Autodesk Inventor part; units mm, degrees
note: some values were not read from the file. Chosen so that the rebuilt part matches the saved one: direction of "Hole2".
(part 2 of 20)
  ellipse E76 centre (-10075.27878, -10011.578305) end of major axis (-10075.513001, -10009.501471) minor radius 0.044517 (-10075.516592, -10009.569699) -> (-10075.486251, -10009.995005) ccw
  ellipse E77 centre (-10074.384652, -10011.477467) end of major axis (-10074.618874, -10009.400632) minor radius 0.044517 (-10074.622381, -10009.471498) -> (-10074.592437, -10009.890575) ccw
  ellipse E78 centre (-10060.476, -10009.908873) end of major axis (-10060.386346, -10010.703833) minor radius 0.01704 (-10060.484477, -10009.985098) -> (-10060.393632, -10010.678018) ccw
  line L94 (-10060.377876, -10010.91364) -> (-10060.484477, -10009.985098)
  ellipse E79 centre (-10059.482525, -10009.79683) end of major axis (-10059.426491, -10010.29368) minor radius 0.01065 (-10059.539194, -10009.3223) -> (-10059.42924, -10010.286086) ccw
  line L95 (-10062.350001, -10017.517567) -> (-10062.806719, -10017.467871)
  line L96 (-10060.454278, -10015.430074) -> (-10060.460552, -10016.580748)
  line L97 (-10059.880259, -10016.422198) -> (-10059.873105, -10015.110144)
  line L98 (-10059.873105, -10015.110144) -> (-10060.046355, -10015.004028)
  ellipse E80 centre (-10060.050028, -10015.677678) end of major axis (-10060.234317, -10014.96604) minor radius 0.371687 (-10060.442629, -10015.281983) -> (-10060.454278, -10015.430074) ccw
  ellipse E81 centre (-10060.050028, -10015.677678) end of major axis (-10060.234317, -10014.96604) minor radius 0.371687 (-10060.046355, -10015.004028) -> (-10060.05419, -10014.999356) ccw
  ellipse E82 centre (-10059.335003, -10016.824224) end of major axis (-10059.248465, -10016.028918) minor radius 0.273562 (-10059.101399, -10016.209395) -> (-10059.155812, -10016.093674) ccw
  line L99 (-10062.350001, -10020.512649) -> (-10062.806719, -10020.562345)
  ellipse E83 centre (-10060.025424, -10022.372531) end of major axis (-10059.932235, -10021.66476) minor radius 0.400382 (-10060.431835, -10022.539755) -> (-10059.992436, -10023.062247) ccw
  line L100 (-10060.063938, -10023.080853) -> (-10060.204432, -10023.096141)
  line L101 (-10060.476356, -10021.608916) -> (-10060.431835, -10022.539755)
  line L102 (-10059.992436, -10023.062247) -> (-10059.81826, -10022.990579)
  line L103 (-10059.81826, -10022.990579) -> (-10059.876504, -10021.77281)
  ellipse E84 centre (-10059.335003, -10021.369758) end of major axis (-10059.248465, -10022.165063) minor radius 0.273562 (-10059.155812, -10022.100307) -> (-10059.101399, -10021.984587) ccw
  ellipse E85 centre (-10061.469475, -10028.173067) end of major axis (-10061.55913, -10028.968027) minor radius 0.01704 (-10061.487267, -10028.178778) -> (-10061.56071, -10028.955341) ccw
  line L104 (-10061.487267, -10028.178778) -> (-10061.380198, -10027.227663)
  ellipse E86 centre (-10059.482525, -10028.397152) end of major axis (-10059.57218, -10029.192112) minor radius 0.01704 (-10059.407624, -10027.670855) -> (-10059.57111, -10029.119451) ccw
  line L105 (-10061.56497, -10026.585239) -> (-10062.078212, -10026.527356)
  ellipse E87 centre (-10075.27878, -10026.615677) end of major axis (-10075.513001, -10028.692511) minor radius 0.044517 (-10075.486251, -10028.198976) -> (-10075.513001, -10028.692511) ccw
  ellipse E88 centre (-10074.384652, -10026.716515) end of major axis (-10074.618874, -10028.793349) minor radius 0.044517 (-10074.592437, -10028.303407) -> (-10074.622381, -10028.722483) ccw
  line L106 (-10060.493792, -10028.290821) -> (-10060.380028, -10027.280229)
  ellipse E89 centre (-10060.476, -10028.285109) end of major axis (-10060.386346, -10027.490149) minor radius 0.01704 (-10060.393632, -10027.515964) -> (-10060.493792, -10028.290821) ccw
  ellipse E90 centre (-10059.482525, -10028.397152) end of major axis (-10059.538559, -10028.894002) minor radius 0.01065 (-10059.427694, -10027.953575) -> (-10059.528515, -10028.845931) ccw
  line L107 (-10061.48836, -10025.278009) -> (-10061.55116, -10026.262694)
  ellipse E91 centre (-10061.350908, -10025.73615) end of major axis (-10061.516786, -10026.518764) minor radius 0.120739 (-10061.55116, -10026.262694) -> (-10061.250304, -10025.840771) ccw
  line L108 (-10061.250304, -10025.840771) -> (-10060.901774, -10024.313165)
  line L109 (-10060.901774, -10024.313165) -> (-10059.934712, -10024.518137)
  ellipse E92 centre (-10059.416785, -10026.146094) end of major axis (-10059.582663, -10026.928708) minor radius 0.120739 (-10059.515377, -10026.862757) -> (-10059.215803, -10025.454922) ccw
  line L110 (-10061.508918, -10026.520431) -> (-10061.516786, -10026.518764)
  line L111 (-10060.925141, -10024.345935) -> (-10060.901774, -10024.313165)
  line L112 (-10060.901774, -10024.313165) -> (-10064.091636, -10023.637063)
  ellipse E93 centre (-10060.325762, -10024.379903) end of major axis (-10060.884685, -10023.567598) minor radius 0.235923 (-10060.180568, -10024.176282) -> (-10060.792125, -10023.567877) ccw
  line L113 (-10061.100929, -10023.500053) -> (-10067.010154, -10022.247573)
  line L114 (-10060.180568, -10024.176282) -> (-10059.934712, -10024.518137)
  line L115 (-10060.283242, -10026.045743) -> (-10059.934712, -10024.518137)
  line L116 (-10061.422518, -10013.14956) -> (-10061.856897, -10013.172389)
  line L117 (-10061.836081, -10012.326253) -> (-10061.553929, -10012.311424)
  line L118 (-10061.409576, -10013.39483) -> (-10061.492385, -10011.825491)
  ellipse E94 centre (-10061.492555, -10011.773328) end of major axis (-10061.534542, -10010.97443) minor radius 0.002573 (-10061.534542, -10010.97443) -> (-10061.492385, -10011.825491) ccw
  line L119 (-10061.36027, -10013.392238) -> (-10061.409576, -10013.39483)
  ellipse E95 centre (-10059.495322, -10011.66836) end of major axis (-10059.537309, -10010.869463) minor radius 0.002573 (-10059.510196, -10011.340621) -> (-10059.515377, -10011.331224) ccw
  line L120 (-10059.537309, -10010.869463) -> (-10061.534542, -10010.97443)
  line L121 (-10061.557698, -10012.065672) -> (-10061.853507, -10012.081219)
  line L122 (-10061.409576, -10013.39483) -> (-10063.048629, -10013.480972)
  ellipse E96 centre (-10059.495322, -10011.66836) end of major axis (-10059.521564, -10011.169049) minor radius 0.001608 (-10059.511461, -10011.338287) -> (-10059.514117, -10011.333468) ccw
  line L123 (-10061.607405, -10010.674865) -> (-10061.68528, -10010.670928)
  line L124 (-10061.783035, -10009.753857) -> (-10061.579243, -10009.76416)
  line L125 (-10061.615601, -10010.939927) -> (-10061.567206, -10009.374897)
  ellipse E97 centre (-10061.420853, -10009.294962) end of major axis (-10061.380459, -10008.495982) minor radius 0.142983 (-10061.380459, -10008.495982) -> (-10061.54092, -10009.012282) ccw
  line L126 (-10061.570957, -10010.942184) -> (-10061.615601, -10010.939927)
  ellipse E98 centre (-10059.455566, -10009.394321) end of major axis (-10059.415172, -10008.595341) minor radius 0.142983 (-10059.342552, -10008.734438) -> (-10059.57111, -10009.07453) ccw
  line L127 (-10059.415172, -10008.595341) -> (-10061.380459, -10008.495982)
  line L128 (-10061.571047, -10009.499098) -> (-10061.816602, -10009.486684)
  line L129 (-10061.615601, -10010.939927) -> (-10061.811814, -10010.930007)
  line L130 (-10063.391932, -10010.850121) -> (-10063.642743, -10010.837441)
  ellipse E99 centre (-10075.079596, -10008.604419) end of major axis (-10074.974067, -10006.517085) minor radius 0.373543 (-10074.974067, -10006.517085) -> (-10075.402988, -10007.952487) ccw
  ellipse E100 centre (-10074.195217, -10008.64913) end of major axis (-10074.089688, -10006.561796) minor radius 0.373543 (-10073.894561, -10006.951244) -> (-10074.51733, -10007.985402) ccw
  line L131 (-10074.974067, -10006.517085) -> (-10074.089688, -10006.561796)
  ellipse E101 centre (-10074.195217, -10008.64913) end of major axis (-10074.119478, -10007.151044) minor radius 0.268093 (-10074.014581, -10007.29359) -> (-10074.41067, -10009.869338) ccw
  ellipse E102 centre (-10059.455566, -10009.394321) end of major axis (-10059.43032, -10008.894959) minor radius 0.089364 (-10059.363417, -10009.208737) -> (-10059.544237, -10009.378772) ccw
  line L132 (-10059.898881, -10015.094356) -> (-10059.801569, -10014.609349)
  line L133 (-10059.801569, -10014.609349) -> (-10059.814039, -10014.600069)
  ellipse E103 centre (-10059.377353, -10016.449287) end of major axis (-10059.172257, -10015.676024) minor radius 0.142054 (-10059.155812, -10016.093674) -> (-10059.172257, -10015.676024) ccw
  line L134 (-10059.172257, -10015.676024) -> (-10059.875174, -10015.489586)
  line L135 (-10062.350001, -10019.545608) -> (-10062.806719, -10019.51725)
  line L136 (-10060.391402, -10027.491423) -> (-10060.332323, -10027.282736)
  ellipse E104 centre (-10060.305787, -10027.725657) end of major axis (-10060.527432, -10028.49434) minor radius 0.14613 (-10060.307433, -10027.284044) -> (-10060.393632, -10027.515964) ccw
  ellipse E105 centre (-10059.361099, -10027.998052) end of major axis (-10059.222572, -10027.517625) minor radius 0.091331 (-10059.227286, -10027.838895) -> (-10059.44944, -10027.974778) ccw
  ellipse E106 centre (-10059.361099, -10027.998052) end of major axis (-10059.139455, -10027.229369) minor radius 0.14613 (-10059.144207, -10027.729902) -> (-10059.407624, -10027.670855) ccw
  line L137 (-10059.139455, -10027.229369) -> (-10059.524741, -10027.118274)
  ellipse E107 centre (-10061.194651, -10025.032179) end of major axis (-10061.48409, -10025.777984) minor radius 0.002457 (-10061.46407, -10025.723867) -> (-10061.48409, -10025.777984) ccw
  ellipse E108 centre (-10061.194651, -10025.032179) end of major axis (-10060.905212, -10024.286374) minor radius 0.002457 (-10061.457945, -10025.707747) -> (-10061.458801, -10025.709998) ccw
  line L138 (-10060.660115, -10023.646866) -> (-10060.655933, -10023.636082)
  line L139 (-10060.655933, -10023.636082) -> (-10059.723681, -10023.997878)
  ellipse E109 centre (-10059.330147, -10025.755773) end of major axis (-10059.040708, -10025.009968) minor radius 0.002457 (-10059.21498, -10025.465271) -> (-10059.215803, -10025.454922) ccw
  line L140 (-10061.474672, -10025.781639) -> (-10061.48409, -10025.777984)
  line L141 (-10059.040708, -10025.009968) -> (-10059.965078, -10024.65123)
  line L142 (-10060.655933, -10023.636082) -> (-10060.696511, -10023.620334)
  line L143 (-10060.883309, -10023.547839) -> (-10065.815027, -10021.633895)
  ellipse E110 centre (-10059.984852, -10023.848112) end of major axis (-10060.377627, -10022.955787) minor radius 0.168714 (-10059.900944, -10023.626312) -> (-10060.345585, -10022.957249) ccw
  line L144 (-10060.345585, -10022.957249) -> (-10064.606408, -10021.303671)
  line L145 (-10059.900944, -10023.626312) -> (-10059.723681, -10023.997878)
  line L146 (-10059.723681, -10023.997878) -> (-10059.956311, -10024.612802)
  line L147 (-10059.947993, -10024.576347) -> (-10059.723681, -10023.997878)
  ellipse E111 centre (-10059.330147, -10025.755773) end of major axis (-10059.149248, -10025.289644) minor radius 0.001536 (-10059.215161, -10025.462782) -> (-10059.215594, -10025.457336) ccw
  line L148 (-10061.167264, -10013.708989) -> (-10061.411584, -10012.430812)
  ellipse E112 centre (-10061.419075, -10012.379718) end of major axis (-10061.569131, -10011.593917) minor radius 0.002231 (-10061.449697, -10012.231033) -> (-10061.411584, -10012.430812) ccw
  ellipse E113 centre (-10061.419075, -10012.379718) end of major axis (-10061.569131, -10011.593917) minor radius 0.002231 (-10061.569131, -10011.593917) -> (-10061.479166, -10012.076002) ccw
  line L149 (-10061.562628, -10011.592675) -> (-10061.569131, -10011.593917)
  line L150 (-10061.435333, -10010.969216) -> (-10061.540297, -10010.029174)
  ellipse E114 centre (-10074.188288, -10011.200402) end of major axis (-10074.334497, -10009.707545) minor radius 0.24157 (-10074.395592, -10009.772988) -> (-10074.425568, -10009.871079) ccw
  ellipse E115 centre (-10074.188288, -10011.200402) end of major axis (-10074.392006, -10009.120355) minor radius 0.336587 (-10074.468892, -10009.193821) -> (-10074.4718, -10009.199795) ccw
  ellipse E116 centre (-10059.45458, -10009.7574) end of major axis (-10059.405844, -10010.255019) minor radius 0.080523 (-10059.453007, -10010.190813) -> (-10059.427468, -10010.241126) ccw
  ellipse E117 centre (-10059.45458, -10009.7574) end of major axis (-10059.503316, -10009.259781) minor radius 0.080523 (-10059.517481, -10009.270082) -> (-10059.543695, -10009.384211) ccw
  ellipse E118 centre (-10061.390902, -10025.808057) end of major axis (-10061.238841, -10025.022641) minor radius 0.086818 (-10061.489391, -10025.861843) -> (-10061.564797, -10026.455678) ccw
  line L151 (-10061.489391, -10025.861843) -> (-10061.456687, -10025.683636)
  line L152 (-10061.230363, -10013.101701) -> (-10061.302045, -10012.860155)
  ellipse E119 centre (-10061.313455, -10012.81413) end of major axis (-10061.540932, -10012.047152) minor radius 0.002152 (-10061.359155, -10012.66747) -> (-10061.302045, -10012.860155) ccw
  ellipse E120 centre (-10061.313455, -10012.81413) end of major axis (-10061.540932, -10012.047152) minor radius 0.002152 (-10061.380234, -10012.596226) -> (-10061.379475, -10012.598795) ccw
  ellipse E121 centre (-10061.313455, -10012.81413) end of major axis (-10061.540932, -10012.047152) minor radius 0.002152 (-10061.540854, -10012.047696) -> (-10061.46729, -10012.301069) ccw
  line L153 (-10059.896065, -10014.082947) -> (-10060.229072, -10014.181713)
  line L154 (-10067.429747, -10016.109617) -> (-10067.426808, -10016.11971)
  line L155 (-10064.222927, -10015.366245) -> (-10067.081482, -10016.214061)
  line L156 (-10059.899344, -10014.071686) -> (-10059.896065, -10014.082947)
  line L157 (-10059.896065, -10014.082947) -> (-10059.936009, -10014.146629)
  line L158 (-10059.896065, -10014.082947) -> (-10059.964617, -10013.851948)
  line L159 (-10061.459654, -10010.510742) -> (-10061.463483, -10010.493181)
  ellipse E122 centre (-10061.347946, -10010.418573) end of major axis (-10061.510562, -10009.635275) minor radius 0.128538 (-10061.5089, -10010.257445) -> (-10061.463483, -10010.493181) ccw
  line L160 (-10060.361849, -10010.912798) -> (-10060.37563, -10010.849592)
  ellipse E123 centre (-10059.415142, -10010.017314) end of major axis (-10059.313507, -10010.506876) minor radius 0.080336 (-10059.449748, -10010.21676) -> (-10059.286923, -10010.372283) ccw
  ellipse E124 centre (-10061.442823, -10028.705225) end of major axis (-10061.437551, -10029.505207) minor radius 0.125799 (-10061.568714, -10028.685033) -> (-10061.437551, -10029.505207) ccw
  line L161 (-10061.568714, -10028.685033) -> (-10061.570469, -10027.970396)
  line L162 (-10061.572527, -10027.132339) -> (-10061.572581, -10027.110703)
  line L163 (-10061.572581, -10027.110703) -> (-10061.543326, -10027.110511)
  ellipse E125 centre (-10059.467748, -10028.69221) end of major axis (-10059.462476, -10029.492193) minor radius 0.125799 (-10059.587131, -10028.407305) -> (-10059.593638, -10028.672019) ccw
  line L164 (-10061.572581, -10027.110703) -> (-10062.110288, -10027.114246)
  line L165 (-10063.114705, -10027.120865) -> (-10063.630156, -10027.124262)
  ellipse E126 centre (-10075.169596, -10028.795676) end of major axis (-10075.155825, -10030.885631) minor radius 0.328649 (-10075.496217, -10028.957967) -> (-10075.432006, -10029.986721) ccw
  ellipse E127 centre (-10074.280812, -10028.789819) end of major axis (-10074.267041, -10030.879774) minor radius 0.328649 (-10074.605637, -10029.03444) -> (-10074.544121, -10029.973038) ccw
  ellipse E128 centre (-10074.280812, -10028.789819) end of major axis (-10074.270929, -10030.289787) minor radius 0.235872 (-10074.507534, -10028.313326) -> (-10074.258015, -10030.287447) ccw
  ellipse E129 centre (-10059.467748, -10028.69221) end of major axis (-10059.464453, -10029.192199) minor radius 0.078624 (-10059.5435, -10028.80781) -> (-10059.40237, -10028.987214) ccw
  ellipse E130 centre (-10061.482864, -10026.278951) end of major axis (-10061.550105, -10027.07612) minor radius 0.002201 (-10061.492125, -10026.362713) -> (-10061.550105, -10027.07612) ccw
  line L166 (-10061.541226, -10027.076869) -> (-10061.550105, -10027.07612)
  line L167 (-10061.167453, -10013.707999) -> (-10064.126659, -10014.257156)
  line L168 (-10061.039851, -10013.929143) -> (-10061.125614, -10013.703446)
  line L169 (-10061.039851, -10013.929143) -> (-10061.318639, -10012.381486)
  ellipse E131 centre (-10061.40265, -10012.352927) end of major axis (-10061.548618, -10011.566356) minor radius 0.077504 (-10061.318639, -10012.381486) -> (-10061.565476, -10011.725973) ccw
  ellipse E132 centre (-10061.40265, -10012.352927) end of major axis (-10061.256682, -10013.139497) minor radius 0.077504 (-10061.565389, -10011.727637) -> (-10061.565107, -10011.732865) ccw
  line L170 (-10061.565107, -10011.732865) -> (-10061.56265, -10011.777155)
  line L171 (-10061.005983, -10013.922858) -> (-10061.039851, -10013.929143)
  line L172 (-10061.514781, -10011.560077) -> (-10061.548618, -10011.566356)
  line L173 (-10061.039851, -10013.929143) -> (-10062.439649, -10014.188911)
  line L174 (-10061.532376, -10011.346389) -> (-10062.092453, -10011.401104)
  line L175 (-10061.413023, -10010.968043) -> (-10061.510032, -10010.0167)
  ellipse E133 centre (-10061.470111, -10009.953691) end of major axis (-10061.547894, -10009.157482) minor radius 0.045982 (-10061.559295, -10009.215401) -> (-10061.510032, -10010.0167) ccw
  line L176 (-10061.568174, -10011.600458) -> (-10062.079075, -10011.650368)
  ellipse E134 centre (-10075.281385, -10011.302921) end of major axis (-10075.484591, -10009.222823) minor radius 0.120129 (-10075.496217, -10009.236015) -> (-10075.502488, -10009.996902) ccw
  ellipse E135 centre (-10074.38713, -10011.215561) end of major axis (-10074.590335, -10009.135463) minor radius 0.120129 (-10074.605637, -10009.159541) -> (-10074.622833, -10009.404086) ccw
  ellipse E136 centre (-10074.38713, -10011.215561) end of major axis (-10074.532971, -10009.722668) minor radius 0.086217 (-10074.479028, -10009.877325) -> (-10074.555987, -10009.886316) ccw
  ellipse E137 centre (-10059.482878, -10009.759558) end of major axis (-10059.531492, -10009.261926) minor radius 0.028739 (-10059.538823, -10009.30312) -> (-10059.539208, -10009.319581) ccw
  line L177 (-10062.093325, -10026.808932) -> (-10061.53368, -10026.863604)
  ellipse E138 centre (-10061.470111, -10028.24029) end of major axis (-10061.547894, -10029.0365) minor radius 0.045982 (-10061.514679, -10028.223624) -> (-10061.559295, -10028.978581) ccw
  line L178 (-10061.514679, -10028.223624) -> (-10061.416311, -10027.225765)
  ellipse E139 centre (-10075.281385, -10026.89106) end of major axis (-10075.484591, -10028.971158) minor radius 0.120129 (-10075.502488, -10028.197079) -> (-10075.496217, -10028.957967) ccw
  ellipse E140 centre (-10074.38713, -10026.978421) end of major axis (-10074.590335, -10029.058518) minor radius 0.120129 (-10074.622833, -10028.789895) -> (-10074.605637, -10029.03444) ccw
  ellipse E141 centre (-10074.38713, -10026.978421) end of major axis (-10074.532971, -10028.471314) minor radius 0.086217 (-10074.555987, -10028.307665) -> (-10074.479028, -10028.316657) ccw
  ellipse E142 centre (-10059.482878, -10028.434424) end of major axis (-10059.434264, -10027.936793) minor radius 0.028739 (-10059.428376, -10027.955754) -> (-10059.44973, -10027.977073) ccw
  ellipse E143 centre (-10059.482878, -10028.434424) end of major axis (-10059.531492, -10028.932055) minor radius 0.028739 (-10059.534008, -10028.71437) -> (-10059.520298, -10028.908651) ccw
  line L179 (-10064.132119, -10023.983552) -> (-10061.199545, -10024.527766)
  ellipse E144 centre (-10061.40265, -10025.841055) end of major axis (-10061.548618, -10026.627626) minor radius 0.077504 (-10061.564797, -10026.455678) -> (-10061.338171, -10025.917057) ccw
  line L180 (-10061.338171, -10025.917057) -> (-10061.052091, -10024.438593)
  line L181 (-10061.514781, -10026.633905) -> (-10061.548618, -10026.627626)
  line L182 (-10061.349313, -10013.521931) -> (-10061.481734, -10011.954571)
  ellipse E145 centre (-10061.482864, -10011.91503) end of major axis (-10061.550105, -10011.117861) minor radius 0.002201 (-10061.491988, -10011.832904) -> (-10061.481734, -10011.954571) ccw
  ellipse E146 centre (-10061.482864, -10011.91503) end of major axis (-10061.550105, -10011.117861) minor radius 0.002201 (-10061.550105, -10011.117861) -> (-10061.492004, -10011.832707) ccw
  line L183 (-10061.205341, -10013.509787) -> (-10061.349313, -10013.521931)
  line L184 (-10061.541226, -10011.117112) -> (-10061.550105, -10011.117861)
  line L185 (-10061.349313, -10013.521931) -> (-10063.058958, -10013.66614)
  line L186 (-10064.155076, -10013.758597) -> (-10064.184618, -10013.761089)
  line L187 (-10061.75465, -10009.995657) -> (-10061.586436, -10009.996765)
  line L188 (-10061.558039, -10011.12484) -> (-10061.568614, -10009.555498)
  ellipse E147 centre (-10061.442823, -10009.488757) end of major axis (-10061.437551, -10008.688774) minor radius 0.125799 (-10061.545763, -10009.055222) -> (-10061.568614, -10009.555498) ccw
  line L189 (-10061.549804, -10011.124894) -> (-10061.558039, -10011.12484)
  line L190 (-10061.558039, -10011.12484) -> (-10062.10792, -10011.121216)
  line L191 (-10063.112778, -10011.114595) -> (-10063.901758, -10011.109396)
  ellipse E148 centre (-10075.169596, -10009.398306) end of major axis (-10075.183368, -10011.48826) minor radius 0.328649 (-10075.432006, -10008.207261) -> (-10075.496217, -10009.236015) ccw
  ellipse E149 centre (-10074.280812, -10009.404162) end of major axis (-10074.294584, -10011.494117) minor radius 0.328649 (-10074.544121, -10008.220944) -> (-10074.605637, -10009.159541) ccw
  ellipse E150 centre (-10074.280812, -10009.404162) end of major axis (-10074.270929, -10007.904195) minor radius 0.235872 (-10074.234932, -10007.922118) -> (-10074.507534, -10009.880655) ccw
  ellipse E151 centre (-10060.455285, -10009.495264) end of major axis (-10060.460557, -10010.295247) minor radius 0.125799 (-10060.581077, -10009.562005) -> (-10060.567785, -10009.883357) ccw
  ellipse E152 centre (-10059.467748, -10009.501772) end of major axis (-10059.464453, -10009.001783) minor radius 0.078624 (-10059.521231, -10009.149201) -> (-10059.5435, -10009.386172) ccw
  line L192 (-10060.370505, -10027.292485) -> (-10060.368084, -10027.280856)
  ellipse E153 centre (-10059.415142, -10028.176667) end of major axis (-10059.313507, -10027.687106) minor radius 0.080336 (-10059.286923, -10027.821699) -> (-10059.449748, -10027.977222) ccw
  ellipse E154 centre (-10061.313455, -10025.379852) end of major axis (-10061.540932, -10026.146829) minor radius 0.002152 (-10061.467677, -10025.894227) -> (-10061.540854, -10026.146286) ccw
  line L193 (-10065.427348, -10022.583054) -> (-10067.278978, -10022.033881)
  line L194 (-10067.427856, -10022.074558) -> (-10067.430593, -10022.084035)
  ellipse E155 centre (-10063.939588, -10011.200613) end of major axis (-10064.143693, -10010.360039) minor radius 0.148059 (-10064.06177, -10011.321594) -> (-10064.04289, -10011.391653) ccw
  ellipse E156 centre (-10063.939588, -10011.200613) end of major axis (-10064.143693, -10010.360039) minor radius 0.148059 (-10064.107684, -10011.13096) -> (-10064.097088, -10011.17798) ccw
  ellipse E157 centre (-10064.75146, -10028.871078) end of major axis (-10064.762971, -10028.414223) minor radius 0.076505 (-10064.803232, -10028.491001) -> (-10064.818056, -10029.04404) ccw
  ellipse E158 centre (-10064.75146, -10028.871078) end of major axis (-10064.729671, -10029.735804) minor radius 0.144806 (-10064.881739, -10028.369511) -> (-10064.650717, -10029.577969) ccw
  ellipse E159 centre (-10065.737035, -10028.895912) end of major axis (-10065.715247, -10029.760637) minor radius 0.144806 (-10065.882555, -10028.678354) -> (-10065.715247, -10029.760637) ccw
  line L195 (-10065.715247, -10029.760637) -> (-10064.729671, -10029.735804)
  ellipse E160 centre (-10064.011809, -10026.154893) end of major axis (-10064.073586, -10027.017684) minor radius 0.002538 (-10064.00735, -10026.057324) -> (-10064.056431, -10026.801617) ccw
  line L196 (-10064.48319, -10026.988356) -> (-10064.073586, -10027.017684)
  ellipse E161 centre (-10063.718913, -10010.220519) end of major axis (-10063.628826, -10011.080815) minor radius 0.036963 (-10063.804797, -10009.36429) -> (-10063.623182, -10011.061534) ccw
  ellipse E162 centre (-10064.712567, -10010.324572) end of major axis (-10064.802654, -10009.464276) minor radius 0.036963 (-10064.802654, -10009.464276) -> (-10064.70624, -10010.704175) ccw
  line L197 (-10064.802654, -10009.464276) -> (-10063.809001, -10009.360223)
  line L198 (-10064.487269, -10011.170709) -> (-10063.628826, -10011.080815)
  ellipse E163 centre (-10063.718913, -10027.973462) end of major axis (-10063.809001, -10028.833758) minor radius 0.036963 (-10063.628765, -10027.113174) -> (-10063.804797, -10028.829692) ccw
  ellipse E164 centre (-10064.712567, -10027.86941) end of major axis (-10064.802654, -10028.729706) minor radius 0.036963 (-10064.70624, -10027.489807) -> (-10064.802654, -10028.729706) ccw
  line L199 (-10064.487269, -10027.023273) -> (-10063.628826, -10027.113166)
  line L200 (-10064.802654, -10028.729706) -> (-10063.809001, -10028.833758)
  ellipse E165 centre (-10064.011809, -10012.039088) end of major axis (-10064.073586, -10011.176297) minor radius 0.002538 (-10064.056431, -10011.392365) -> (-10064.00735, -10012.136657) ccw
  line L201 (-10064.48319, -10011.205626) -> (-10064.073586, -10011.176297)
  ellipse E166 centre (-10064.75146, -10009.322903) end of major axis (-10064.739948, -10008.866048) minor radius 0.076505 (-10064.818056, -10009.149942) -> (-10064.803232, -10009.70298) ccw
  ellipse E167 centre (-10064.75146, -10009.322903) end of major axis (-10064.729671, -10008.458178) minor radius 0.144806 (-10064.650717, -10008.616013) -> (-10064.881739, -10009.824471) ccw
  ellipse E168 centre (-10065.737035, -10009.29807) end of major axis (-10065.715247, -10008.433344) minor radius 0.144806 (-10065.715247, -10008.433344) -> (-10065.882555, -10009.515627) ccw
  line L202 (-10065.715247, -10008.433344) -> (-10064.729671, -10008.458178)
  ellipse E169 centre (-10061.974755, -10012.635827) end of major axis (-10061.876064, -10013.082043) minor radius 0.001467 (-10062.048245, -10012.30816) -> (-10061.878293, -10013.070431) ccw
  ellipse E170 centre (-10061.974755, -10012.635827) end of major axis (-10062.161554, -10011.791238) minor radius 0.002777 (-10062.06806, -10012.225192) -> (-10061.82596, -10013.316212) ccw
  ellipse E171 centre (-10062.951154, -10012.851779) end of major axis (-10063.137953, -10012.007189) minor radius 0.002777 (-10063.113287, -10012.125264) -> (-10062.824847, -10013.432208) ccw
  line L203 (-10062.960663, -10009.32244) -> (-10062.85822, -10009.31082)
  line L204 (-10062.960663, -10028.871541) -> (-10062.85822, -10028.883162)
  ellipse E172 centre (-10061.974755, -10025.558155) end of major axis (-10061.876064, -10025.111938) minor radius 0.001467 (-10061.878293, -10025.123551) -> (-10062.048245, -10025.885822) ccw
  ellipse E173 centre (-10061.974755, -10025.558155) end of major axis (-10061.787956, -10024.713566) minor radius 0.002777 (-10061.85943, -10025.026728) -> (-10062.06806, -10025.96879) ccw
  ellipse E174 centre (-10062.951154, -10025.342203) end of major axis (-10062.764354, -10024.497614) minor radius 0.002777 (-10062.865532, -10024.943732) -> (-10063.113287, -10026.068718) ccw
  ellipse E175 centre (-10061.84899, -10012.626786) end of major axis (-10061.949329, -10012.180937) minor radius 0.077418 (-10061.821582, -10012.427374) -> (-10061.794928, -10013.029999) ccw
  ellipse E176 centre (-10061.84899, -10012.626786) end of major axis (-10062.03891, -10011.782893) minor radius 0.146534 (-10061.875117, -10013.084798) -> (-10061.844696, -10013.171748) ccw
  ellipse E177 centre (-10061.84899, -10012.626786) end of major axis (-10062.03891, -10011.782893) minor radius 0.146534 (-10061.821554, -10012.172715) -> (-10062.070758, -10011.823837) ccw
  line L205 (-10062.071752, -10011.790284) -> (-10062.03891, -10011.782893)
  ellipse E178 centre (-10061.84899, -10025.567196) end of major axis (-10061.949329, -10026.013044) minor radius 0.077418 (-10061.791574, -10025.158469) -> (-10061.796905, -10025.680045) ccw
  ellipse E179 centre (-10061.84899, -10025.567196) end of major axis (-10061.659071, -10024.723302) minor radius 0.146534 (-10061.86776, -10025.087351) -> (-10061.875117, -10025.109184) ccw
  ellipse E180 centre (-10061.84899, -10025.567196) end of major axis (-10062.03891, -10026.411089) minor radius 0.146534 (-10062.070758, -10026.370144) -> (-10061.758405, -10025.810623) ccw
  line L206 (-10062.071752, -10026.403698) -> (-10062.03891, -10026.411089)
  ellipse E181 centre (-10062.995762, -10013.860793) end of major axis (-10063.308717, -10013.054392) minor radius 0.002657 (-10063.065996, -10013.686988) -> (-10062.930843, -10014.035241) ccw
  ellipse E182 centre (-10063.928014, -10014.22259) end of major axis (-10064.240969, -10013.416188) minor radius 0.002657 (-10064.050328, -10013.914199) -> (-10063.931504, -10014.220939) ccw
  ellipse E183 centre (-10063.13135, -10011.283056) end of major axis (-10063.371003, -10010.451917) minor radius 0.158003 (-10063.330798, -10011.148517) -> (-10063.276026, -10011.35135) ccw
  ellipse E184 centre (-10063.13135, -10011.283056) end of major axis (-10063.371003, -10010.451917) minor radius 0.158003 (-10063.404768, -10010.757439) -> (-10063.34361, -10011.094898) ccw
  ellipse E185 centre (-10062.955742, -10028.976619) end of major axis (-10062.932667, -10029.433036) minor radius 0.081679 (-10063.037774, -10028.749134) -> (-10062.880488, -10028.880636) ccw
  ellipse E186 centre (-10062.955742, -10028.976619) end of major axis (-10062.912066, -10029.840515) minor radius 0.1546 (-10063.108614, -10028.506472) -> (-10062.80578, -10028.892844) ccw
  ellipse E187 centre (-10063.938385, -10029.026298) end of major axis (-10063.894709, -10029.890195) minor radius 0.1546 (-10064.098844, -10028.803407) -> (-10063.894709, -10029.890195) ccw
  line L207 (-10063.894709, -10029.890195) -> (-10062.912066, -10029.840515)
  ellipse E188 centre (-10062.07375, -10026.390109) end of major axis (-10062.097735, -10026.846479) minor radius 0.00147 (-10062.052277, -10025.995625) -> (-10062.060503, -10026.162324) ccw
  ellipse E189 centre (-10062.07375, -10026.390109) end of major axis (-10062.119149, -10027.253916) minor radius 0.002783 (-10062.0495, -10025.885666) -> (-10062.071679, -10026.403714) ccw
  ellipse E190 centre (-10063.072367, -10026.337625) end of major axis (-10063.026968, -10025.473817) minor radius 0.002783 (-10063.034751, -10025.594831) -> (-10063.04342, -10025.748101) ccw
  ellipse E191 centre (-10063.072367, -10026.337625) end of major axis (-10063.117765, -10027.201433) minor radius 0.002783 (-10063.048248, -10025.835565) -> (-10063.117765, -10027.201433) ccw
  line L208 (-10063.117765, -10027.201433) -> (-10062.119149, -10027.253916)
  ellipse E192 centre (-10063.267625, -10012.864086) end of major axis (-10063.08827, -10013.710288) minor radius 0.130549 (-10063.08827, -10013.710288) -> (-10063.44698, -10012.017885) ccw
  ellipse E193 centre (-10064.234687, -10013.069058) end of major axis (-10064.055331, -10013.91526) minor radius 0.130549 (-10064.149355, -10013.802914) -> (-10064.359442, -10012.264782) ccw
  line L209 (-10064.365541, -10012.212577) -> (-10063.44698, -10012.017885)
  line L210 (-10064.055331, -10013.91526) -> (-10063.08827, -10013.710288)
  ellipse E194 centre (-10061.766525, -10010.054416) end of major axis (-10061.81774, -10009.600294) minor radius 0.009734
  ellipse E195 centre (-10061.766525, -10010.054416) end of major axis (-10061.669586, -10010.913967) minor radius 0.018424 (-10061.684102, -10010.670988) -> (-10061.667872, -10010.898405) ccw
  ellipse E196 centre (-10062.76, -10010.166458) end of major axis (-10062.663061, -10011.026009) minor radius 0.018424 (-10062.856938, -10009.306907) -> (-10062.676115, -10010.969337) ccw
  line L211 (-10062.856938, -10009.306907) -> (-10061.863463, -10009.194865)
  line L212 (-10062.117209, -10010.964449) -> (-10061.669586, -10010.913967)
  ellipse E197 centre (-10061.766525, -10028.139566) end of major axis (-10061.81774, -10028.593687) minor radius 0.009734
  ellipse E198 centre (-10061.766525, -10028.139566) end of major axis (-10061.863463, -10028.999117) minor radius 0.018424 (-10061.671655, -10027.283395) -> (-10061.686547, -10027.549722) ccw
  ellipse E199 centre (-10062.76, -10028.027524) end of major axis (-10062.856938, -10028.887075) minor radius 0.018424 (-10062.676115, -10027.224644) -> (-10062.856938, -10028.887075) ccw
  line L213 (-10062.856938, -10028.887075) -> (-10061.863463, -10028.999117)
  ellipse E200 centre (-10063.267625, -10025.329895) end of major axis (-10063.44698, -10026.176097) minor radius 0.130549 (-10063.44698, -10026.176097) -> (-10063.08827, -10024.483694) ccw
  ellipse E201 centre (-10064.234687, -10025.124923) end of major axis (-10064.414042, -10025.971125) minor radius 0.130549 (-10064.359442, -10025.9292) -> (-10064.102151, -10024.309896) ccw
  line L214 (-10064.055331, -10024.278722) -> (-10063.08827, -10024.483694)
  line L215 (-10064.365541, -10025.981405) -> (-10063.44698, -10026.176097)
  ellipse E202 centre (-10062.07375, -10011.803873) end of major axis (-10062.049765, -10012.260243) minor radius 0.00147 (-10062.060503, -10012.031657) -> (-10062.052277, -10012.198356) ccw
  ellipse E203 centre (-10062.07375, -10011.803873) end of major axis (-10062.119149, -10010.940065) minor radius 0.002783 (-10062.071679, -10011.790268) -> (-10062.0495, -10012.308315) ccw
  ellipse E204 centre (-10063.072367, -10011.856357) end of major axis (-10063.117765, -10010.992549) minor radius 0.002783 (-10063.04342, -10012.44588) -> (-10063.034751, -10012.59915) ccw
  ellipse E205 centre (-10063.072367, -10011.856357) end of major axis (-10063.117765, -10010.992549) minor radius 0.002783 (-10063.117765, -10010.992549) -> (-10063.048248, -10012.358417) ccw
  line L216 (-10063.117765, -10010.992549) -> (-10062.119149, -10010.940065)
  ellipse E206 centre (-10062.955742, -10009.217363) end of major axis (-10062.932667, -10008.760946) minor radius 0.081679 (-10062.880488, -10009.313346) -> (-10063.037774, -10009.444848) ccw
  ellipse E207 centre (-10062.955742, -10009.217363) end of major axis (-10062.912066, -10008.353466) minor radius 0.1546 (-10062.80578, -10009.301138) -> (-10063.108614, -10009.687509) ccw
  ellipse E208 centre (-10063.938385, -10009.167684) end of major axis (-10063.894709, -10008.303787) minor radius 0.1546 (-10063.894709, -10008.303787) -> (-10064.098844, -10009.390575) ccw
  line L217 (-10063.894709, -10008.303787) -> (-10062.912066, -10008.353466)
  ellipse E209 centre (-10063.13135, -10026.910926) end of major axis (-10062.891697, -10026.079787) minor radius 0.158003 (-10063.276026, -10026.842632) -> (-10063.29728, -10026.917123) ccw
  ellipse E210 centre (-10062.995762, -10024.333188) end of major axis (-10062.682806, -10023.526787) minor radius 0.002657 (-10062.948154, -10024.203267) -> (-10062.999959, -10024.336662) ccw
  ellipse E211 centre (-10063.928014, -10023.971392) end of major axis (-10063.615058, -10023.16499) minor radius 0.002657 (-10063.948782, -10024.017575) -> (-10064.021801, -10024.206034) ccw
  ellipse E212 centre (-10067.605233, -10010.542508) end of major axis (-10067.688487, -10009.681524) minor radius 0.221488 (-10067.821941, -10009.961734) -> (-10067.832883, -10010.057822) ccw
  ellipse E213 centre (-10067.605233, -10027.651474) end of major axis (-10067.521978, -10026.79049) minor radius 0.221488 (-10067.832883, -10028.13616) -> (-10067.821941, -10028.232248) ccw
  ellipse E214 centre (-10066.598757, -10028.739199) end of major axis (-10066.601768, -10028.282209) minor radius 0.071862 (-10066.668171, -10028.601607) -> (-10066.662683, -10028.93188) ccw
  ellipse E215 centre (-10066.598757, -10028.739199) end of major axis (-10066.593057, -10029.60418) minor radius 0.13602 (-10066.733807, -10028.595195) -> (-10066.600713, -10029.602863) ccw
  ellipse E216 centre (-10067.586295, -10028.745706) end of major axis (-10067.580595, -10029.610688) minor radius 0.13602 (-10067.688781, -10028.150237) -> (-10067.595304, -10029.605735) ccw
  ellipse E217 centre (-10065.688015, -10010.36574) end of major axis (-10065.732448, -10009.910906) minor radius 0.026267 (-10065.729401, -10009.913235) -> (-10065.735003, -10009.913822) ccw
  ellipse E218 centre (-10065.688015, -10010.36574) end of major axis (-10065.772117, -10009.504839) minor radius 0.049718 (-10065.763375, -10009.514609) -> (-10065.718791, -10010.550723) ccw
  ellipse E219 centre (-10066.681631, -10010.462807) end of major axis (-10066.765733, -10009.601905) minor radius 0.049718 (-10066.765733, -10009.601905) -> (-10066.737914, -10010.396275) ccw
  line L218 (-10066.765733, -10009.601905) -> (-10065.772117, -10009.504839)
  ellipse E220 centre (-10065.688015, -10027.828241) end of major axis (-10065.732448, -10028.283076) minor radius 0.026267 (-10065.735003, -10028.280159) -> (-10065.729401, -10028.280746) ccw
  ellipse E221 centre (-10065.688015, -10027.828241) end of major axis (-10065.772117, -10028.689143) minor radius 0.049718 (-10065.718791, -10027.643259) -> (-10065.763375, -10028.679373) ccw
  ellipse E222 centre (-10066.681631, -10027.731174) end of major axis (-10066.765733, -10028.592076) minor radius 0.049718 (-10066.737914, -10027.797706) -> (-10066.765733, -10028.592076) ccw
  line L219 (-10066.765733, -10028.592076) -> (-10065.772117, -10028.689143)
  ellipse E223 centre (-10066.598757, -10009.454783) end of major axis (-10066.595746, -10008.997792) minor radius 0.071862 (-10066.662683, -10009.262101) -> (-10066.668171, -10009.592375) ccw
  ellipse E224 centre (-10066.598757, -10009.454783) end of major axis (-10066.593057, -10008.589801) minor radius 0.13602 (-10066.600713, -10008.591119) -> (-10066.733807, -10009.598787) ccw
  ellipse E225 centre (-10067.586295, -10009.448275) end of major axis (-10067.580595, -10008.583294) minor radius 0.13602 (-10067.595304, -10008.588247) -> (-10067.688781, -10010.043745) ccw
  ellipse E226 centre (-10139.4756, -10019.096991) end of major axis (-10140.215912, -10019.031075) minor radius 0.194882 (-10139.697274, -10018.891991) -> (-10139.253927, -10019.301991) ccw
  line L220 (-10137.244268, -10019.301991) -> (-10139.253927, -10019.301991)
  line L221 (-10137.687031, -10018.891991) -> (-10139.697274, -10018.891991)
  ellipse E227 centre (-10139.476021, -10016.96267) end of major axis (-10140.230129, -10016.819513) minor radius 0.195462 (-10139.676479, -10016.735578) -> (-10140.005713, -10017.01046) ccw
  line L222 (-10117.710141, -10019.446062) -> (-10118.514279, -10019.361928)
  line L223 (-10138.134367, -10016.896923) -> (-10139.676479, -10016.735578)
  ellipse E228 centre (-10139.476021, -10021.231311) end of major axis (-10140.243423, -10021.247408) minor radius 0.195482 (-10140.226791, -10021.205538) -> (-10139.233127, -10021.412017) ccw
  line L224 (-10138.228313, -10021.306888) -> (-10139.233127, -10021.412017)
  line L225 (-10117.710141, -10018.74792) -> (-10118.514279, -10018.832053)
  ellipse E229 centre (-10137.46565, -10019.096991) end of major axis (-10138.20264, -10019.030826) minor radius 0.194809 (-10137.687031, -10018.891991) -> (-10137.244268, -10019.301991) ccw
  line L226 (-10120.709018, -10019.301991) -> (-10137.244268, -10019.301991)
  line L227 (-10120.709018, -10018.891991) -> (-10137.687031, -10018.891991)
  ellipse E230 centre (-10137.465514, -10016.931519) end of major axis (-10138.217838, -10016.779288) minor radius 0.195466 (-10137.663174, -10016.70203) -> (-10137.930242, -10017.000562) ccw
  line L228 (-10110.696072, -10020.265564) -> (-10117.710307, -10019.446045)
  line L229 (-10119.021168, -10018.880099) -> (-10137.663174, -10016.70203)
  line L230 (-10110.694219, -10019.301991) -> (-10117.198671, -10019.301991)
  line L231 (-10110.694219, -10018.891991) -> (-10117.198671, -10018.891991)
  ellipse E231 centre (-10137.465514, -10021.262463) end of major axis (-10138.232664, -10021.287802) minor radius 0.195478 (-10138.192506, -10021.222449) -> (-10137.220414, -10021.440221) ccw
  line L232 (-10119.021168, -10019.313882) -> (-10137.220414, -10021.440221)
  line L233 (-10110.696072, -10017.928417) -> (-10117.710307, -10018.747937)
  ellipse E232 centre (-10141.503707, -10019.096991) end of major axis (-10142.268604, -10019.033112) minor radius 0.195472 (-10141.726593, -10018.891991) -> (-10141.280821, -10019.301991) ccw
  line L234 (-10141.259793, -10019.301991) -> (-10141.280821, -10019.301991)
  line L235 (-10141.703573, -10018.891991) -> (-10141.726593, -10018.891991)
  ellipse E233 centre (-10141.481683, -10019.096991) end of major axis (-10142.22464, -10019.031277) minor radius 0.19494 (-10141.703573, -10018.891991) -> (-10141.259793, -10019.301991) ccw
  line L236 (-10139.253927, -10019.301991) -> (-10141.259793, -10019.301991)
  line L237 (-10139.697274, -10018.891991) -> (-10141.703573, -10018.891991)
  ellipse E234 centre (-10141.482508, -10016.97894) end of major axis (-10142.237965, -10016.843154) minor radius 0.195467 (-10141.685106, -10016.753818) -> (-10141.279909, -10017.204063) ccw
  ellipse E235 centre (-10110.685615, -10019.898058) end of major axis (-10110.66627, -10019.693973) minor radius 0.000002 (-10110.66627, -10019.693973) -> (-10110.689578, -10019.939846) ccw
  line L238 (-10118.513381, -10019.362014) -> (-10119.02126, -10019.313874)
  line L239 (-10123.472153, -10018.891991) -> (-10141.279909, -10017.204063)
  line L240 (-10110.66627, -10019.693973) -> (-10114.801709, -10019.301991)
  line L241 (-10140.196001, -10016.894965) -> (-10141.685106, -10016.753818)
  ellipse E236 centre (-10141.482508, -10021.215041) end of major axis (-10142.250021, -10021.223641) minor radius 0.195476 (-10141.723692, -10021.031983) -> (-10141.241324, -10021.398099) ccw
  ellipse E237 centre (-10110.685615, -10018.295923) end of major axis (-10110.66627, -10018.500009) minor radius 0.000002 (-10110.689578, -10018.254136) -> (-10110.66627, -10018.500009) ccw
  line L242 (-10110.66627, -10018.500009) -> (-10114.801709, -10018.891991)
  line L243 (-10140.212637, -10021.300594) -> (-10141.241324, -10021.398099)
  line L244 (-10118.513381, -10018.831968) -> (-10119.02126, -10018.880108)
  line L245 (-10123.472153, -10019.301991) -> (-10141.723692, -10021.031983)
  line L246 (-10067.949916, -10028.148973) -> (-10067.964876, -10028.123265)
  line L247 (-10068.069898, -10028.207417) -> (-10068.068326, -10028.200288)
  line L248 (-10068.054556, -10028.233781) -> (-10068.069898, -10028.207417)
  line L249 (-10068.069898, -10028.207417) -> (-10068.099808, -10028.204322)
  line L250 (-10068.102422, -10029.81232) -> (-10068.101613, -10029.795011)
  line L251 (-10068.101613, -10029.795011) -> (-10068.121454, -10029.747612)
  line L252 (-10068.164781, -10029.644109) -> (-10068.178644, -10029.610993)
  line L253 (-10068.250286, -10029.439846) -> (-10068.260394, -10029.4157)
  line L254 (-10068.269418, -10029.608908) -> (-10068.260394, -10029.4157)
  line L255 (-10068.235225, -10029.690591) -> (-10068.269418, -10029.608908)
  line L256 (-10068.260394, -10029.4157) -> (-10068.261639, -10029.415731)
  line L257 (-10068.269418, -10029.608908) -> (-10068.325933, -10029.610332)
  line L258 (-10070.169747, -10029.65679) -> (-10070.1701, -10029.656799)
  line L259 (-10072.263733, -10029.709552) -> (-10072.288547, -10029.710177)
  line L260 (-10068.321328, -10029.045143) -> (-10068.305795, -10029.082249)
  line L261 (-10068.334378, -10029.045472) -> (-10068.321328, -10029.045143)
  line L262 (-10068.321328, -10029.045143) -> (-10068.315842, -10028.927692)
  line L263 (-10068.308841, -10028.777793) -> (-10068.286227, -10028.29362)
  line L264 (-10068.238925, -10009.861648) -> (-10068.241185, -10009.834738)
  line L265 (-10068.26163, -10009.591224) -> (-10068.262363, -10009.582495)
  line L266 (-10068.325675, -10009.32737) -> (-10068.318485, -10009.301983)
  line L267 (-10068.320701, -10009.38662) -> (-10068.325675, -10009.32737)
  line L268 (-10068.325675, -10009.32737) -> (-10068.344345, -10009.3269)
  line L269 (-10068.368496, -10008.906779) -> (-10068.275009, -10008.909134)
  line L270 (-10068.289805, -10008.732908) -> (-10068.275009, -10008.909134)
  line L271 (-10072.310399, -10008.631601) -> (-10072.292134, -10008.632062)
  line L272 (-10070.190487, -10008.685017) -> (-10070.169283, -10008.685551)
  line L273 (-10068.356997, -10008.731215) -> (-10068.289805, -10008.732908)
  line L274 (-10068.275009, -10008.909134) -> (-10068.239925, -10008.785261)
  line L275 (-10068.15993, -10008.502817) -> (-10068.156254, -10008.489837)
  line L276 (-10068.289805, -10008.732908) -> (-10068.244918, -10008.574421)
  line L277 (-10068.069933, -10008.424404) -> (-10068.075167, -10008.442883)
  line L278 (-10068.216063, -10009.96621) -> (-10068.21375, -10009.953355)
  line L279 (-10067.995835, -10029.747088) -> (-10068.003465, -10029.972626)
  line L280 (-10067.965046, -10030.060587) -> (-10068.003465, -10029.972626)
  line L281 (-10067.954368, -10029.744991) -> (-10067.965046, -10030.060587)
  line L282 (-10067.965046, -10030.060587) -> (-10068.011927, -10030.062957)
  line L283 (-10068.056905, -10030.270354) -> (-10068.050463, -10030.079949)
  line L284 (-10068.111835, -10030.273131) -> (-10068.056905, -10030.270354)
  line L285 (-10068.050463, -10030.079949) -> (-10068.227925, -10029.673653)
  line L286 (-10068.234367, -10029.864058) -> (-10068.227925, -10029.673653)
  line L287 (-10068.056905, -10030.270354) -> (-10068.234367, -10029.864058)
  line L288 (-10068.227925, -10029.673653) -> (-10068.234345, -10029.673978)
  line L289 (-10068.234367, -10029.864058) -> (-10068.243819, -10029.864536)
  line L290 (-10072.303275, -10029.496472) -> (-10072.272871, -10029.494935)
  line L291 (-10068.251636, -10009.176766) -> (-10068.251813, -10009.17369)
  line L292 (-10068.264197, -10008.958267) -> (-10068.267574, -10008.899512)
  line L293 (-10068.305126, -10009.006623) -> (-10068.267574, -10008.899512)
  line L294 (-10068.301922, -10009.062355) -> (-10068.305126, -10009.006623)
  line L295 (-10068.267574, -10008.899512) -> (-10068.272218, -10008.899277)
  line L296 (-10068.305126, -10009.006623) -> (-10068.362924, -10009.003701)
  line L297 (-10070.188279, -10008.911417) -> (-10070.200153, -10008.910817)
  line L298 (-10068.243134, -10008.598181) -> (-10068.239095, -10008.598385)
  line L299 (-10068.249461, -10008.418056) -> (-10068.239095, -10008.598385)
  line L300 (-10068.268562, -10008.417091) -> (-10068.249461, -10008.418056)
  line L301 (-10068.239095, -10008.598385) -> (-10068.065643, -10008.103633)
  line L302 (-10068.076009, -10007.923305) -> (-10068.065643, -10008.103633)
  line L303 (-10068.249461, -10008.418056) -> (-10068.076009, -10007.923305)
  line L304 (-10068.076009, -10007.923305) -> (-10068.128796, -10007.920636)
  line L305 (-10067.977892, -10008.073226) -> (-10068.015443, -10008.180337)
  line L306 (-10068.026855, -10008.07075) -> (-10067.977892, -10008.073226)
  line L307 (-10068.015443, -10008.180337) -> (-10068.000133, -10008.446677)
  line L308 (-10067.977892, -10008.073226) -> (-10067.956297, -10008.448893)
  line L309 (-10068.266229, -10029.232122) -> (-10068.287844, -10029.165208)
  line L310 (-10068.301325, -10029.353281) -> (-10068.287844, -10029.165208)
  line L311 (-10068.266526, -10029.461013) -> (-10068.301325, -10029.353281)
  line L312 (-10068.287844, -10029.165208) -> (-10068.338441, -10029.165542)
  line L313 (-10070.191036, -10029.177749) -> (-10070.613505, -10029.180533)
  line L314 (-10068.301325, -10029.353281) -> (-10068.344802, -10029.353567)
  line L315 (-10070.199818, -10029.365791) -> (-10070.205792, -10029.36583)
  line L316 (-10072.303174, -10029.379651) -> (-10072.329925, -10029.379827)
  line L317 (-10068.246022, -10010.098182) -> (-10068.306531, -10009.373218)
  line L318 (-10068.33587, -10009.477432) -> (-10068.306531, -10009.373218)
  line L319 (-10068.31283, -10009.753472) -> (-10068.33587, -10009.477432)
  line L320 (-10068.306531, -10009.373218) -> (-10068.316424, -10009.373153)
  line L321 (-10068.33587, -10009.477432) -> (-10068.358073, -10009.477286)
  line L322 (-10072.333528, -10009.45109) -> (-10072.364524, -10009.450886)
  line L323 (-10086.460185, -10026.52999) -> (-10086.564188, -10027.525223)
  line L324 (-10087.359355, -10030.323681) -> (-10087.061474, -10027.473194)
  ellipse E238 centre (-10087.133995, -10028.170574) end of major axis (-10087.39414, -10030.657003) minor radius 0.000177 (-10087.359355, -10030.323681) -> (-10087.39414, -10030.657003) ccw
  line L325 (-10085.506151, -10030.854535) -> (-10087.39414, -10030.657003)
  line L326 (-10086.564188, -10010.668759) -> (-10086.460185, -10011.663992)
  line L327 (-10087.061474, -10010.720788) -> (-10087.359355, -10007.870301)
  ellipse E239 centre (-10087.133995, -10010.023407) end of major axis (-10087.39414, -10007.536979) minor radius 0.000177 (-10087.39414, -10007.536979) -> (-10087.359355, -10007.870301) ccw
  line L328 (-10087.39414, -10007.536979) -> (-10085.506151, -10007.339447)
  ellipse E240 centre (-10082.643707, -10027.896583) end of major axis (-10082.672719, -10028.144894) minor radius 0.000013
  ellipse E241 centre (-10082.518842, -10026.828138) end of major axis (-10082.588111, -10027.421005) minor radius 0.00003 (-10082.582182, -10027.37016) -> (-10082.582158, -10027.370162) ccw
  ellipse E242 centre (-10082.926301, -10030.317146) end of major axis (-10082.833946, -10029.526678) minor radius 0.000039 (-10082.967167, -10030.666626) -> (-10082.96711, -10030.666733) ccw